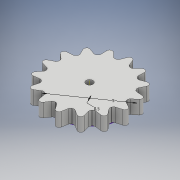
# Autodesk Inventor part: gear
Saved by Autodesk Inventor 2018 (Build 220112000, 112)
## iProperties
Created: 2019-02-11
Part Number: gear
Material: Genérico
Document SubType Name: Modeling
Designer: EDWIN
Density: 1 g/cm^3
Appearance: Valor por defecto
Author: EDWIN
Autodesk Inventor part; units mm, degrees
ref_plane "YZ Plane" through (0, 0, 0) normal (1, 0, 0) x (0, 1, 0)
ref_plane "XZ Plane" through (0, 0, 0) normal (0, 1, 0) x (-1, 0, 0)
ref_plane "XY Plane" through (0, 0, 0) normal (0, 0, 1) x (1, 0, 0)
sketch "Boceto1" plane through (0, 0, 0) normal (0, 0, 1) x (1, 0, 0)
  circle A0 centre (0, 0) radius 2.5
  circle A1 centre (0, 0) radius 0.25
  dimension "d0" = 5
  dimension "d12" = 0.5
  constraints: 2 centre point, 2 coincident
  measures "d0" diameter of A0
  measures "d12" diameter of A1
extrude "Extrusión1" add sketch "Boceto1" along normal blind 1 contours A0 | A1
sketch "Boceto2" plane through (0, 0, 1) normal (0, 0, 1) x (1, 0, 0)
  line L0 (-0.125, 3.1279) -> (0.125, 3.1279)
  line L1 (-0.5, 2.2) -> (0.5, 2.2)
  line L2 (-0.125, 3.1279) -> (-0.5, 2.2)
  line L3 (0.5, 2.2) -> (0.125, 3.1279)
  line L4 (0, 0) -> (0, 2.2)
  point P0 (0, 3.1279)
  point P1 (0, 2.2)
  dimension "d3" = 0.25
  dimension "d4" = 1
  dimension "d5" = 2.2
  constraints: 10 end point, 2 horizontal, 2 midpoint, 1 vertical, 1 vertical alignment
  measures "d3" distance of L0.start L0.end
  measures "d4" distance of L1.start L1.end
  measures "d5" distance of L4.start L4.end
extrude "Extrusión2" add sketch "Boceto2" against normal blind 1
fillet "Empalme1" radius 0.2 4 edges at (0.125, 3.1279, 0.5) (-0.125, 3.1279, 0.5) (-0.3912, 2.4692, 0.5) (0.3912, 2.4692, 0.5)
pattern_circular "Patrón circular1" count 15 over 360 about axis through (0, 0, 0) along (0, 0, 1) of "Empalme1", "Extrusión2"
extrude "Extrusión3" cut sketch "Boceto1" along normal blind 1 contours A1
